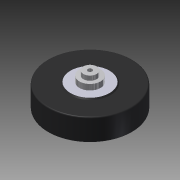
# Autodesk Inventor part: Roue
Saved by Autodesk Inventor 2016 (Build 200138000, 138)
## iProperties
Created: 2015-10-02
Part Number: Roue
Material: Générique
Document SubType Name: Modeling
Designer: Logan
Density: 1 g/cm^3
Appearance: Par défaut
Author: Logan
Autodesk Inventor part; units mm, degrees
ref_plane "YZ Plane" through (0, 0, 0) normal (1, 0, 0) x (0, 1, 0)
ref_plane "XZ Plane" through (0, 0, 0) normal (0, 1, 0) x (-1, 0, 0)
ref_plane "XY Plane" through (0, 0, 0) normal (0, 0, 1) x (1, 0, 0)
sketch "Esquisse1" plane through (0, 0, 0) normal (0, 0, 1) x (1, 0, 0)
  circle A0 centre (0, 0) radius 38.1
  circle A1 centre (0, 0) radius 2
  dimension "d0" = 76.2
  dimension "d1" = 4
  constraints: 2 centre point, 2 coincident
  measures "d0" diameter of A0
  measures "d1" diameter of A1
extrude "Extrusion1" add sketch "Esquisse1" along normal blind 20
sketch "Esquisse2" plane through (0, 0, 20) normal (0, 0, 1) x (1, 0, 0)
  circle A0 centre (0, 0) radius 2 projected
  circle A1 centre (0, 0) radius 38.1 projected
  circle A2 centre (0, 0) radius 17.7233
  constraints: 1 centre point
extrude "Extrusion2" add sketch "Esquisse2" along normal blind 1 and the other way blind 21 contours A2
fillet "Congé1" radius 1 2 edges at (-38.1, 0, 20) (-38.1, 0, 0)
chamfer "Chanfrein1" distance 1 angle 45 2 edges at (-17.7233, 0, 20) (-17.7233, 0, 0)
sketch "Esquisse3" plane through (0, 0, -1) normal (0, 0, -1) x (-1, 0, 0)
  circle A0 centre (0, 0) radius 2 projected
  circle A1 centre (0, 0) radius 17.7233 projected
  circle A2 centre (0, 0) radius 16.7233
  circle A3 centre (0, 0) radius 3
  dimension "d12" = 1
  dimension "d13" = 1
  constraints: 2 centre point
  measures "d12" radial gap between concentric circles of A1 A2
  measures "d13" radial gap between concentric circles of A0 A3
extrude "Extrusion3" cut sketch "Esquisse3" against normal blind 1 contours A2
sketch "Esquisse4" plane through (0, 0, 21) normal (0, 0, 1) x (1, 0, 0)
  circle A0 centre (0, 0) radius 9.6
  circle A1 centre (0, 0) radius 2 projected
  circle A2 centre (0, 0) radius 17.7233 projected
  dimension "d16" = 19.2
  constraints: 1 centre point, 1 coincident
  measures "d16" diameter of A0
extrude "Extrusion4" add sketch "Esquisse4" along normal blind 5.1 contours A0
sketch "Esquisse5" plane through (0, 0, 26.1) normal (0, 0, 1) x (1, 0, 0)
  circle A0 centre (0, 0) radius 2 projected
  circle A1 centre (0, 0) radius 9.6 projected
  circle A2 centre (0, 0) radius 6.05
  dimension "d19" = 12.1
  constraints: 1 centre point, 1 coincident
  measures "d19" diameter of A2
extrude "Extrusion5" add sketch "Esquisse5" along normal blind 4.1 contours A2
